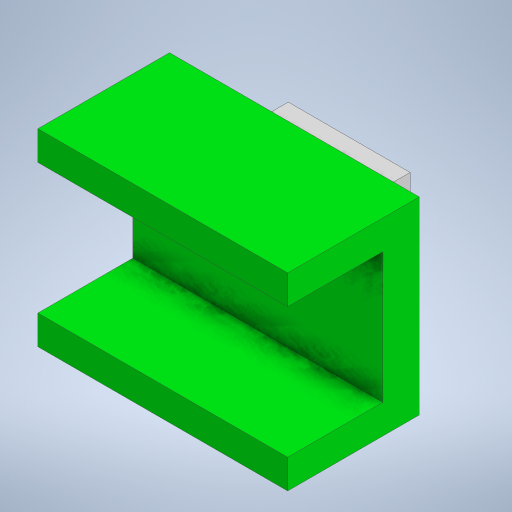
# Autodesk Inventor part: 스텝모터 드라이버
Saved by Autodesk Inventor 2023 (Build 270158000, 158)
## iProperties
Created: 2022-11-11
Part Number: 스텝모터 드라이버
Material: 일반
Document SubType Name: Modeling
Designer: hyunsu
Density: 1 g/cm^3
Appearance: 기본값
Author: hyunsu
Autodesk Inventor part; units mm, degrees
ref_plane "YZ Plane" through (0, 0, 0) normal (1, 0, 0) x (0, 1, 0)
ref_plane "XZ Plane" through (0, 0, 0) normal (0, 1, 0) x (-1, 0, 0)
ref_plane "XY Plane" through (0, 0, 0) normal (0, 0, 1) x (1, 0, 0)
sketch "스케치1" plane through (0, 0, 0) normal (0, 0, 1) x (1, 0, 0)
  line L0 (-10.25, -7.75) -> (10.25, -7.75)
  line L1 (10.25, -7.75) -> (10.25, 7.75)
  line L2 (10.25, 7.75) -> (-10.25, 7.75)
  line L3 (-10.25, 7.75) -> (-10.25, -7.75)
  line L4 (-10.25, -7.75) -> (10.25, 7.75) construction
  line L5 (10.25, -7.75) -> (-10.25, 7.75) construction
  point P0 (0, 0)
  dimension "d0" = 20.5
  dimension "d1" = 15.5
  constraints: 12 end point, 2 midpoint, 2 parallel, 1 horizontal, 1 perpendicular
  measures "d0" distance of L2.end L1.end
  measures "d1" distance of L1.end L0.end
extrude "돌출1" add sketch "스케치1" along normal blind 3
sketch "스케치2" plane through (0, 0, 3) normal (0, 0, 1) x (1, 0, 0)
  line L0 (10.25, 7.75) -> (-10.25, 7.75) projected
  line L1 (-10.25, 7.75) -> (10.25, 7.75)
  line L2 (10.25, 7.75) -> (10.25, 5.35)
  line L3 (10.25, 5.35) -> (-10.25, 5.35)
  line L4 (-10.25, 5.35) -> (-10.25, 7.75)
  line L5 (0, 0) -> (4.2226, 0)
  line L6 (10.25, -7.75) -> (-10.25, -7.75)
  line L7 (-10.25, -7.75) -> (10.25, -7.75)
  line L8 (10.25, -7.75) -> (10.25, -5.35)
  line L9 (10.25, -5.35) -> (-10.25, -5.35)
  line L10 (-10.25, -5.35) -> (-10.25, -7.75)
  dimension "d4" = 2.4
  constraints: 20 end point, 5 symmetric about line, 2 horizontal, 2 parallel, 1 perpendicular
  measures "d4" distance between parallel lines of L0 L3
extrude "돌출2" add sketch "스케치2" along normal blind 7.8
sketch "스케치3" plane through (0, 0, 0) normal (0, 0, -1) x (-1, 0, 0)
  line L0 (-5, -5.3868) -> (5, -5.3868)
  line L1 (5, -5.3868) -> (5, 4.6132)
  line L2 (5, 4.6132) -> (-5, 4.6132)
  line L3 (-5, 4.6132) -> (-5, -5.3868)
  line L4 (-5, -5.3868) -> (5, 4.6132) construction
  line L5 (5, -5.3868) -> (-5, 4.6132) construction
  point P0 (0, 0)
  point P1 (0, -0.3868)
  dimension "d7" = 10
  dimension "d8" = 10
  constraints: 12 end point, 2 midpoint, 2 parallel, 1 horizontal, 1 perpendicular
  measures "d7" distance of L2.end L1.end
  measures "d8" distance of L1.end L0.end
extrude "돌출3" add sketch "스케치3" along normal blind 4.5
